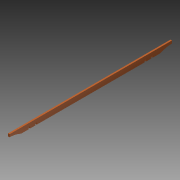
# Autodesk Inventor part: Cover Board
Saved by Autodesk Inventor 2016 (Build 200138000, 138)
## iProperties
Created: 2014-06-08
Part Number: Cover Board
Material: Wood (Cherry)
Document SubType Name: Modeling
Designer: Haden
Density: 0.63 g/cm^3
Appearance: Cherry - Natural Low Gloss
Author: Haden
Autodesk Inventor part; units mm, degrees
ref_plane "YZ Plane" through (0, 0, 0) normal (1, 0, 0) x (0, 1, 0)
ref_plane "XZ Plane" through (0, 0, 0) normal (0, 1, 0) x (-1, 0, 0)
ref_plane "XY Plane" through (0, 0, 0) normal (0, 0, 1) x (1, 0, 0)
sketch "Sketch1" plane through (0, 0, 0) normal (0, 0, 1) x (1, 0, 0)
  line L0 (0, 0) -> (38.1, 0)
  line L1 (38.1, 0) -> (38.1, -139.7)
  line L2 (38.1, -139.7) -> (0, -139.7)
  line L3 (0, -139.7) -> (0, 0)
  dimension "d0" = 38.1
  dimension "d1" = 139.7
  constraints: 8 end point, 2 parallel, 1 horizontal, 1 perpendicular
  measures "d0" distance of L1.end L2.end
  measures "d1" distance of L0.end L1.end
extrude "Extrusion1" add sketch "Sketch1" along normal blind 4267.2
sketch "Sketch2" plane through (38.1, -139.7, 0) normal (1, 0, 0) x (0, 0, -1)
  line L0 (0, 139.7) -> (0, 0) projected
  line L1 (0, 139.7) -> (-4267.2, 139.7) projected
  line L2 (-4267.2, 0) -> (-4267.2, 139.7) projected
  line L3 (0, 0) -> (-4267.2, 0) projected
  line L4 (-4267.2, 139.7) -> (-4267.2, 0) projected
  line L5 (0, 0) -> (-4267.2, 0) projected
  line L6 (-4267.2, 0) -> (-4267.2, 139.7) projected
  arc A0 (-3962.4, 0) -> (-4267.2, 69.85) centre (-4267.2, -630.0932) ccw
  line L7 (0, 0) -> (-4267.2, 0) projected
  line L8 (0, 0) -> (0, 139.7) projected
  arc A1 (0, 69.85) -> (-304.8, 0) centre (0, -630.0932) ccw
  line L9 (-3765.55, 0) -> (-3765.55, 50.8)
  line L10 (-3765.55, 50.8) -> (-3727.45, 50.8)
  line L11 (-3727.45, 50.8) -> (-3727.45, 0)
  line L12 (-3587.75, 0) -> (-3587.75, 50.8)
  line L13 (-3587.75, 50.8) -> (-3549.65, 50.8)
  line L14 (-717.55, 0) -> (-717.55, 50.8)
  line L15 (-717.55, 50.8) -> (-679.45, 50.8)
  line L16 (-679.45, 50.8) -> (-679.45, 0)
  line L17 (-539.75, 0) -> (-539.75, 50.8)
  line L18 (-539.75, 50.8) -> (-501.65, 50.8)
  line L19 (-501.65, 50.8) -> (-501.65, 0)
  line L20 (-3549.65, 50.8) -> (-3549.65, 0)
  dimension "d8" = 304.8
  dimension "d9" = 304.8
  dimension "d12" = 38.1
  dimension "d13" = 50.8
  dimension "d14" = 139.7
  dimension "d15" = 501.65
  dimension "d16" = 139.7
  dimension "d17" = 501.65
  constraints: 24 end point, 8 perpendicular, 6 collinear, 4 point on circle, 4 vertical, 2 centre point, 2 midpoint, 2 vertical alignment, 11 other
  measures "d8" distance from line of A0.start L2
  measures "d9" distance from line of L0 A1.end
  measures "d12" distance of L17.end L18.end
  measures "d13" distance of L18.end L19.end
  measures "d14" distance between parallel lines of L16 L17
  measures "d15" distance between parallel lines of L0 L19
  measures "d16" distance between parallel lines of L11 L12
  measures "d17" distance between parallel lines of L4 L9
extrude "Extrusion2" cut sketch "Sketch2" along normal through all both and the other way through all contours L0 L3 A1 | A0 L3 L2 | L3 L17 L18 L19 | L9 L10 L11 L3 | L3 L14 L15 L16 | L12 L13 L20 L3
body "Solid1"
